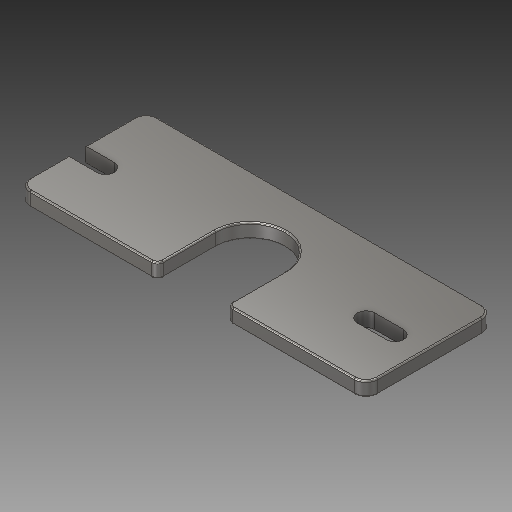
# Autodesk Inventor part: Extruder Plate
Saved by Autodesk Inventor 2020.2 (Build 242310000, 310)
## iProperties
Created: 2018-08-21
Part Number: Extruder Plate
Material: Stainless Steel
Document SubType Name: Modeling
Designer: Richard
Density: 8 g/cm^3
Appearance: Semi-Polished
Author: Richard
Title: J-Head Hotend Extruder Mounting Plate
Autodesk Inventor part; units mm, degrees
ref_plane "YZ Plane" through (0, 0, 0) normal (1, 0, 0) x (0, 1, 0)
ref_plane "XZ Plane" through (0, 0, 0) normal (0, 1, 0) x (-1, 0, 0)
ref_plane "XY Plane" through (0, 0, 0) normal (0, 0, 1) x (1, 0, 0)
sketch "Sketch1" plane through (0, 0, 0) normal (0, 1, 0) x (-1, 0, 0)
  line L0 (-30, 11) -> (-6, 11)
  line L1 (30, 11) -> (30, 2.5)
  line L2 (30, -11) -> (-30, -11)
  line L3 (-30, -11) -> (-30, 11)
  line L4 (-30, 11) -> (30, -11) construction
  line L5 (30, 11) -> (-30, -11) construction
  line L6 (6, 11) -> (6, 1)
  line L7 (-6, 1) -> (-6, 11)
  arc A0 (-6, 1) -> (6, 1) centre (0, 1) ccw
  line L8 (-20, 1) -> (-25, 1) construction
  line L9 (-20, 2.5) -> (-25, 2.5)
  line L10 (-25, -0.5) -> (-20, -0.5)
  arc A1 (-20, -0.5) -> (-20, 2.5) centre (-20, 1) ccw
  arc A2 (-25, 2.5) -> (-25, -0.5) centre (-25, 1) ccw
  line L11 (30, 1) -> (25, 1) construction
  line L12 (30, 2.5) -> (25, 2.5)
  line L13 (25, -0.5) -> (30, -0.5)
  arc A3 (30, -0.5) -> (30, 2.5) centre (30, 1) ccw construction
  arc A4 (25, 2.5) -> (25, -0.5) centre (25, 1) ccw
  line L14 (30, -0.5) -> (30, -11)
  line L15 (30, 2.5) -> (30, -0.5) construction
  line L16 (6, 11) -> (30, 11)
  line L17 (-6, 11) -> (6, 11) construction
  point P0 (0, 0)
  point P1 (0, 0)
  point P2 (0, 0)
  point P3 (-22.5, 1)
  point P4 (27.5, 1)
  dimension "d0" = 60
  dimension "d1" = 22
  dimension "d3" = 1
  dimension "d4" = 12
  dimension "d5" = 5
  dimension "d6" = 3
  dimension "d7" = 10
  dimension "d8" = 5
  dimension "d9" = 5
  constraints: 40 end point, 12 perpendicular, 10 point on circle, 10 tangent, 9 parallel, 6 midpoint, 5 centre point, 4 horizontal, 1 collinear, 1 equal radius, 1 vertical, 1 vertical alignment
  measures "d0" distance of L2.start L2.end
  measures "d1" distance of L1.start L2.start
  measures "d3" distance of point (0, 0) A0.centre
  measures "d4" distance between parallel lines of L7 L6
  measures "d5" distance of L8.start L8.end
  measures "d6" distance between parallel lines of L9 L10
  measures "d7" distance between parallel lines of L0 L8
  measures "d8" distance from line of L3 L8.end
  measures "d9" distance from line of L13.start L1
extrude "Extrusion1" add sketch "Sketch1" along normal mid plane 2.5
fillet "Fillet1" radius 2 4 edges at (-30, 0, -11) (-30, 0, 11) (30, 0, -11) (30, 0, 11)
fillet "Fillet1" radius 1 2 edges at (-6, 0, 11) (6, 0, 11)
fillet "Fillet2" radius 0.25 30 edges at (0, 1.25, -5) (6, 1.25, 5.5) (6.2929, 1.25, 10.7071) (17.5, 1.25, 11) (29.4142, 1.25, 10.4142) (30, 1.25, 0) (29.4142, 1.25, -10.4142) (0, 1.25, -11) (-29.4142, 1.25, -10.4142) (-30, 1.25, -4.75) (-6.2929, 1.25, 10.7071) (-17.5, 1.25, 11) (-29.4142, 1.25, 10.4142) (-30, 1.25, 5.75) (-6, 1.25, 5.5) (-6.2929, -1.25, 10.7071) (-17.5, -1.25, 11) (-29.4142, -1.25, 10.4142) (-30, -1.25, 5.75) (0, -1.25, -5) (6, -1.25, 5.5) (6.2929, -1.25, 10.7071) (17.5, -1.25, 11) (29.4142, -1.25, 10.4142) (30, -1.25, 0) (29.4142, -1.25, -10.4142) (0, -1.25, -11) (-29.4142, -1.25, -10.4142) (-30, -1.25, -4.75) (-6, -1.25, 5.5)
equation "\"d8\" = d5"
body "Solid1"
